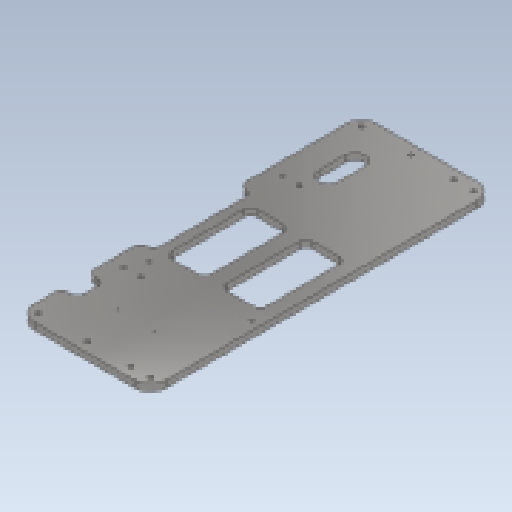
# Autodesk Inventor part: Support_plate
Saved by Autodesk Inventor 2025.2 (Build 292293000, 293)
## iProperties
Created: 2025-02-20
Part Number: Support_plate
Material: Stainless Steel
Document SubType Name: Modeling
Designer: Sergio Quintero
Density: 8 g/cm^3
Appearance: Semi-Polished
Mass: 8245.1 g
Surface Area: 2223.4 cm^2
Volume: 1030.64 cm^3
Author: Sergio Quintero
Autodesk Inventor part; units mm, degrees
note: some values were not read from the file. Chosen so that the rebuilt part matches the saved one: pattern direction of "Rectangular Pattern1".
ref_plane "YZ Plane" through (0, 0, 0) normal (1, 0, 0) x (0, 1, 0)
ref_plane "XZ Plane" through (0, 0, 0) normal (0, 1, 0) x (-1, 0, 0)
ref_plane "XY Plane" through (0, 0, 0) normal (0, 0, 1) x (1, 0, 0)
sketch "Sketch1" plane through (0, 0, 0) normal (0, 1, 0) x (-1, 0, 0)
  line L0 (-100, -260) -> (100, -260)
  line L1 (100, -260) -> (100, 260)
  line L2 (100, 260) -> (-100, 260)
  line L3 (-100, 260) -> (-100, -260)
  line L4 (-100, -260) -> (100, 260) construction
  line L5 (100, -260) -> (-100, 260) construction
  point P0 (0, 0)
  dimension "d0" = 200
  dimension "d1" = 520
  constraints: 12 end point, 2 midpoint, 2 parallel, 1 horizontal, 1 perpendicular
  measures "d0" distance of L2.end L1.end
  measures "d1" distance of L1.end L0.end
extrude "Extrusion1" add sketch "Sketch1" along normal blind 10
fillet "Fillet1" radius 25 4 edges at (-100, 5, -260) (-100, 5, 260) (100, 5, 260) (100, 5, -260)
sketch "Sketch2" plane through (0, 10, 0) normal (0, 1, 0) x (1, 0, 0)
  line L0 (100, -235) -> (100, 235) projected
  line L1 (-75, -260) -> (75, -260) projected
  point P0 (0, 0)
  point P1 (85, -245)
  dimension "d5" = 15
  dimension "d6" = 15
  measures "d5" distance from line of L0 point (85, -245)
  measures "d6" distance from line of point (85, -245) L1
hole "Hole1" at (85, 10, 245) direction (0, -1, 0) diameter 6.647 end through all thread size "M8x1.25" class "6H" standard "ISO Metric profile"
pattern_linear "Rectangular Pattern1" count 2 spacing 170 along (-1, 0, 0) count 2 spacing 490 along (0, 0, -1) of "Hole1"
sketch "Sketch3" plane through (0, 10, 0) normal (0, 1, 0) x (1, 0, 0)
  line L0 (-75, -260) -> (75, -260) projected
  line L1 (-100, 235) -> (-100, -235) projected
  point P0 (0, 0)
  point P1 (-10, -245)
  point P2 (55, -245)
  dimension "d20" = 15
  dimension "d21" = 90
  dimension "d22" = 65
  dimension "d23" = 15
  measures "d20" distance from line of L0 point (-10, -245)
  measures "d21" distance from line of L1 point (-10, -245)
  measures "d22" distance of point (-10, -245) point (55, -245)
  measures "d23" distance from line of L0 point (55, -245)
hole "Hole2" at (-10, 10, 245) at (55, 10, 245) direction (0, -1, 0) diameter 6.647 end through all thread size "M8x1.25" class "6H" standard "ISO Metric profile"
mirror "Mirror1" about plane through (0, 0, 0) normal (0, 0, 1) of "Hole2"
sketch "Sketch12" plane through (0, 10, 0) normal (0, 1, 0) x (1, 0, 0)
  line L0 (-75, -260) -> (75, -260) projected
  line L1 (-100, 235) -> (-100, -235) projected
  point P0 (0, 0)
  point P1 (-55, -120)
  point P2 (-80, -120)
  dimension "d109" = 140
  dimension "d110" = 140
  dimension "d111" = 20
  dimension "d112" = 25
  measures "d109" distance from line of L0 point (-55, -120)
  measures "d110" distance from line of L0 point (-80, -120)
  measures "d111" distance from line of L1 point (-80, -120)
  measures "d112" distance of point (-80, -120) point (-55, -120)
hole "Hole8" at (-55, 10, 120) at (-80, 10, 120) direction (0, -1, 0) diameter 6.647 depth 22.2 tip angle 118 thread size "M8x1.25" class "6H" standard "ISO Metric profile"
mirror "Mirror3" about plane through (0, 0, 0) normal (0, 0, 1) of "Hole8"
sketch "Sketch13" plane through (0, 10, 0) normal (0, 1, 0) x (1, 0, 0)
  line L0 (-100, 235) -> (-100, -235) projected
  line L1 (-100, 75) -> (-80, 75)
  line L2 (-80, 75) -> (-80, -75)
  line L3 (-80, -75) -> (-100, -75)
  line L4 (-100, -75) -> (-100, 75)
  line L5 (0, 0) -> (-146.667, 0) construction
  dimension "d120" = 20
  dimension "d121" = 150
  constraints: 10 end point, 2 horizontal, 2 parallel, 1 perpendicular, 1 point on line, 1 other
  measures "d120" distance of L2.end L3.end
  measures "d121" distance of L1.end L2.end
extrude "Extrusion5" cut sketch "Sketch13" against normal through all
fillet "Fillet5" radius 10 4 edges at (-100, 5, -75) (-100, 5, 75) (-80, 5, 75) (-80, 5, -75)
sketch "Sketch14" plane through (0, 10, 0) normal (0, 1, 0) x (1, 0, 0)
  line L0 (94, -98) -> (-76, -98) construction
  line L1 (-76, -98) -> (-76, -88) construction
  line L2 (-76, -88) -> (94, -88) construction
  line L3 (94, -88) -> (94, -98) construction
  line L4 (94, -98) -> (-76, -88) construction
  line L5 (-76, -98) -> (94, -88) construction
  line L6 (-75, -260) -> (75, -260) construction
  line L7 (100, -235) -> (100, 235) construction
  line L8 (9, -88) -> (9, -98) construction
  point P0 (0, 0)
  point P1 (9, -93)
  point P2 (-69, -93)
  point P3 (87, -93)
  point P4 (-76, -93)
  dimension "d125" = 170
  dimension "d126" = 10
  dimension "d127" = 172
  dimension "d128" = 6
  dimension "d129" = 7
  dimension "d130" = 5
  constraints: 14 end point, 5 midpoint, 2 parallel, 1 horizontal, 1 perpendicular, 1 symmetric about line
  measures "d125" distance of L1.end L2.end
  measures "d126" distance of L0.end L1.end
  measures "d127" distance between parallel lines of L6 L2
  measures "d128" distance between parallel lines of L7 L3
  measures "d129" distance of point (-76, -93) point (-69, -93)
  measures "d130" distance from line of L2 point (-69, -93)
hole "Hole9" at (-69, 10, 93) at (87, 10, 93) direction (0, -1, 0) diameter 4.917 end through all thread size "M6x1" class "6H" standard "ISO Metric profile"
sketch "Sketch8" plane through (0, 10, 0) normal (0, 1, 0) x (1, 0, 0)
  line L0 (-100, 235) -> (-100, -235) projected
  line L1 (-100, -155) -> (-75, -155)
  line L2 (-75, -155) -> (-75, -195)
  line L3 (-75, -195) -> (-100, -195)
  line L4 (-100, -195) -> (-100, -155)
  line L5 (-75, -260) -> (75, -260) projected
  point P0 (0, 0)
  dimension "d72" = 25
  dimension "d73" = 40
  dimension "d74" = 65
  constraints: 8 end point, 2 parallel, 1 horizontal, 1 perpendicular, 1 point on line
  measures "d72" distance of L2.end L3.end
  measures "d73" distance of L1.end L2.end
  measures "d74" distance between parallel lines of L5 L3
extrude "Extrusion2" cut sketch "Sketch8" against normal blind 10
fillet "Fillet2" radius 10 4 edges at (-100, 5, 155) (-75, 5, 155) (-100, 5, 195) (-75, 5, 195)
sketch "Sketch10" plane through (0, 10, 0) normal (0, 1, 0) x (1, 0, 0)
  line L0 (-30, 210) -> (-60, 210)
  line L1 (-60, 210) -> (-60, 140)
  line L2 (-60, 140) -> (-30, 140)
  line L3 (-30, 140) -> (-30, 210)
  line L4 (-100, 235) -> (-100, -145) projected
  line L5 (75, 260) -> (-75, 260) projected
  point P0 (0, 0)
  dimension "d85" = 30
  dimension "d86" = 70
  dimension "d87" = 40
  dimension "d154" = 120
  constraints: 8 end point, 2 parallel, 1 horizontal, 1 perpendicular
  measures "d85" distance of L2.end L1.end
  measures "d86" distance of L1.end L0.end
  measures "d87" distance between parallel lines of L4 L1
  measures "d154" distance between parallel lines of L2 L5
extrude "Extrusion4" cut sketch "Sketch10" against normal blind 10
fillet "Fillet4" radius 15 4 edges at (-60, 5, -140) (-60, 5, -210) (-30, 5, -210) (-30, 5, -140)
sketch "Sketch15" plane through (0, 10, 0) normal (0, 1, 0) x (1, 0, 0)
  line L0 (93, 83.1) -> (-75, 83.1) construction
  line L1 (-75, 83.1) -> (-75, -88.1) construction
  line L2 (-75, -88.1) -> (93, -88.1) construction
  line L3 (93, -88.1) -> (93, 83.1) construction
  line L4 (93, 83.1) -> (-75, -88.1) construction
  line L5 (-75, 83.1) -> (93, -88.1) construction
  line L6 (-80, 65) -> (-80, -65) construction
  line L7 (-5, 57) -> (-65, 57)
  line L8 (-65, 57) -> (-65, -73)
  line L9 (-65, -73) -> (-5, -73)
  line L10 (-5, -73) -> (-5, 57)
  line L11 (19, -73) -> (79, -73)
  line L12 (79, -73) -> (79, 57)
  line L13 (79, 57) -> (19, 57)
  line L14 (19, 57) -> (19, -73)
  point P0 (0, 0)
  point P1 (9, -2.5)
  dimension "d140" = 168
  dimension "d141" = 171.2
  dimension "d142" = 5
  dimension "d143" = 2.5
  dimension "d144" = 26.1
  dimension "d145" = 10
  dimension "d146" = 15.1
  dimension "d147" = 70
  dimension "d148" = 14
  dimension "d149" = 74
  dimension "d150" = 24
  constraints: 28 end point, 6 parallel, 3 horizontal, 3 perpendicular, 2 collinear, 2 midpoint
  measures "d140" distance of L2.end L1.end
  measures "d141" distance of L1.end L0.end
  measures "d142" distance between parallel lines of L1 L6
  measures "d143" vertical distance of point (0, 0) point (9, -2.5)
  measures "d144" distance between parallel lines of L0 L7
  measures "d145" distance between parallel lines of L1 L8
  measures "d146" distance between parallel lines of L2 L9
  measures "d147" distance between parallel lines of L10 L1
  measures "d148" distance between parallel lines of L3 L12
  measures "d149" distance between parallel lines of L14 L3
  measures "d150" distance between parallel lines of L14 L10
extrude "Extrusion6" cut sketch "Sketch15" against normal blind 10
fillet "Fillet6" radius 10 8 edges at (-65, 5, -57) (19, 5, -57) (-5, 5, -57) (79, 5, -57) (-65, 5, 73) (19, 5, 73) (79, 5, 73) (-5, 5, 73)
sketch "Sketch16" plane through (0, 10, 0) normal (0, 1, 0) x (1, 0, 0)
  line L0 (-75, -260) -> (75, -260) projected
  line L1 (100, -235) -> (100, 235) projected
  point P0 (0, 0)
  point P1 (26, -180)
  point P2 (-29, -180)
  dimension "d155" = 80
  dimension "d156" = 80
  dimension "d157" = 55
  dimension "d158" = 74
  measures "d155" distance from line of L0 point (26, -180)
  measures "d156" distance from line of L0 point (-29, -180)
  measures "d157" distance of point (26, -180) point (-29, -180)
  measures "d158" distance from line of L1 point (26, -180)
hole "Hole10" at (26, 10, 180) at (-29, 10, 180) direction (0, -1, 0) diameter 2.459 end through all thread size "M3x0.5" class "6H" standard "ISO Metric profile"
sketch "Sketch11" plane through (0, 10, 0) normal (0, 1, 0) x (1, 0, 0)
  line L0 (-100, 235) -> (-100, -145) projected
  line L1 (-100, -205) -> (-100, -235) projected
  line L2 (75, 260) -> (-75, 260) projected
  line L3 (-75, -260) -> (75, -260) projected
  point P0 (0, 0)
  point P1 (-50, 220)
  point P2 (-50, 70)
  point P3 (-50, -80)
  point P4 (-50, -155)
  point P5 (-50, -230)
  dimension "d92" = 50
  dimension "d93" = 50
  dimension "d94" = 50
  dimension "d95" = 50
  dimension "d96" = 50
  dimension "d97" = 40
  dimension "d98" = 190
  dimension "d99" = 180
  dimension "d100" = 105
  dimension "d101" = 30
  measures "d92" distance from line of L0 point (-50, 220)
  measures "d93" distance from line of L0 point (-50, 70)
  measures "d94" distance from line of L0 point (-50, -80)
  measures "d95" distance from line of L0 point (-50, -155)
  measures "d96" distance from line of L1 point (-50, -230)
  measures "d97" distance from line of L2 point (-50, 220)
  measures "d98" distance from line of L2 point (-50, 70)
  measures "d99" distance from line of L3 point (-50, -80)
  measures "d100" distance from line of L3 point (-50, -155)
  measures "d101" distance from line of L3 point (-50, -230)
body "Solid1"
